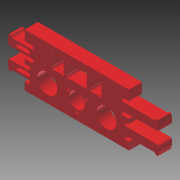
# Autodesk Inventor part: gantry6
Saved by Autodesk Inventor 2012 SP1 (Build 160190100, 190)
## iProperties
Created: 2011-10-14
Part Number: gantry6
Document SubType Name: Modeling
Designer: cramera
Density: 0.952 g/cm^3
Material: High Density Polyethylene
Mass: 43.3758 g
Surface Area: 190.421 cm^2
Volume: 45.5628 cm^3
Autodesk Inventor part; units mm, degrees
ref_plane "YZ Plane" through (0, 0, 0) normal (1, 0, 0) x (0, 1, 0)
ref_plane "XZ Plane" through (0, 0, 0) normal (0, 1, 0) x (-1, 0, 0)
ref_plane "XY Plane" through (0, 0, 0) normal (0, 0, 1) x (1, 0, 0)
derived "skeleton.ipt"
sketch "DRILL-THROUGH" plane through (0, 0, 0) normal (0, 0, 1) x (1, 0, 0)
  arc A0 (91.9322, 359.304) -> (93.4322, 360.804) centre (91.9322, 360.804) ccw
  arc A1 (93.4322, 360.804) -> (91.9322, 362.304) centre (91.9322, 360.804) ccw
  arc A2 (91.9322, 362.304) -> (90.4322, 360.804) centre (91.9322, 360.804) ccw
  arc A3 (90.4322, 360.804) -> (91.9322, 359.304) centre (91.9322, 360.804) ccw
  arc A4 (75.4345, 359.304) -> (76.9345, 360.804) centre (75.4345, 360.804) ccw
  arc A5 (76.9345, 360.804) -> (75.4345, 362.304) centre (75.4345, 360.804) ccw
  arc A6 (75.4345, 362.304) -> (73.9345, 360.804) centre (75.4345, 360.804) ccw
  arc A7 (73.9345, 360.804) -> (75.4345, 359.304) centre (75.4345, 360.804) ccw
  arc A8 (83.6834, 345.0165) -> (85.1834, 346.5165) centre (83.6834, 346.5165) ccw
  arc A9 (85.1834, 346.5165) -> (83.6834, 348.0165) centre (83.6834, 346.5165) ccw
  arc A10 (83.6834, 348.0165) -> (82.1834, 346.5165) centre (83.6834, 346.5165) ccw
  arc A11 (82.1834, 346.5165) -> (83.6834, 345.0165) centre (83.6834, 346.5165) ccw
  constraints: 24 point on circle, 12 centre point
sketch "STOCK_12MM" plane through (0, 0, 0) normal (0, 0, 1) x (1, 0, 0)
  line L0 (914.4, 914.4) -> (457.2, 914.4)
  line L1 (457.2, 914.4) -> (457.2, 0)
  line L2 (0, 0) -> (457.2, 0)
  line L3 (457.2, 0) -> (457.2, 914.4)
  line L4 (457.2, 914.4) -> (0, 914.4)
  line L5 (0, 914.4) -> (0, 0)
  line L6 (457.2, 0) -> (914.4, 0)
  line L7 (914.4, 0) -> (914.4, 914.4)
  constraints: 16 end point
sketch "THROUGH-CUT" plane through (0, 0, 0) normal (0, 0, 1) x (1, 0, 0)
  arc A0 (74.7934, 371.8768) -> (77.0384, 369.6317) centre (75.9159, 370.7543) ccw
  line L0 (77.0384, 369.6317) -> (90.3283, 369.6317)
  arc A1 (90.3283, 369.6317) -> (92.5734, 369.6317) centre (91.4508, 370.7543) ccw
  arc A2 (92.5734, 369.6317) -> (92.5734, 371.8768) centre (91.4508, 370.7543) ccw
  line L1 (92.5734, 371.8768) -> (92.5734, 379.7057)
  arc A3 (92.5734, 379.7057) -> (90.3283, 381.9507) centre (91.4508, 380.8282) ccw
  line L2 (90.3283, 381.9507) -> (77.0384, 381.9507)
  arc A4 (77.0384, 381.9507) -> (74.7934, 379.7057) centre (75.9159, 380.8282) ccw
  line L3 (74.7934, 379.7057) -> (74.7934, 371.8768)
  arc A5 (95.8754, 371.8768) -> (98.1204, 369.6317) centre (96.9979, 370.7543) ccw
  line L4 (98.1204, 369.6317) -> (103.7903, 369.6317)
  arc A6 (103.7903, 369.6317) -> (106.0354, 369.6317) centre (104.9128, 370.7543) ccw
  arc A7 (106.0354, 369.6317) -> (106.0354, 371.8768) centre (104.9128, 370.7543) ccw
  line L5 (106.0354, 371.8768) -> (106.0354, 379.7057)
  arc A8 (106.0354, 379.7057) -> (103.7903, 381.9507) centre (104.9128, 380.8282) ccw
  line L6 (103.7903, 381.9507) -> (98.1204, 381.9507)
  arc A9 (98.1204, 381.9507) -> (95.8754, 379.7057) centre (96.9979, 380.8282) ccw
  line L7 (95.8754, 379.7057) -> (95.8754, 371.8768)
  arc A10 (69.2463, 369.6317) -> (71.4914, 371.8768) centre (70.3688, 370.7543) ccw
  line L8 (71.4914, 371.8768) -> (71.4914, 379.7057)
  arc A11 (71.4914, 379.7057) -> (69.2463, 381.9507) centre (70.3688, 380.8282) ccw
  line L9 (69.2463, 381.9507) -> (63.5764, 381.9507)
  arc A12 (63.5764, 381.9507) -> (61.3314, 379.7057) centre (62.4539, 380.8282) ccw
  line L10 (61.3314, 379.7057) -> (61.3314, 371.8768)
  arc A13 (61.3314, 371.8768) -> (61.3314, 369.6317) centre (62.4539, 370.7543) ccw
  arc A14 (61.3314, 369.6317) -> (63.5764, 369.6317) centre (62.4539, 370.7543) ccw
  line L11 (63.5764, 369.6317) -> (69.2463, 369.6317)
  circle A15 centre (83.6834, 356.0415) radius 7.1882
  circle A16 centre (56.6971, 356.0411) radius 9.04
  circle A17 centre (110.6721, 356.0411) radius 9.04
  arc A18 (39.2334, 370.5512) -> (40.8209, 372.1387) centre (39.2334, 372.1387) ccw
  line L12 (40.8209, 372.1387) -> (40.8209, 372.2657)
  arc A19 (40.8209, 372.2657) -> (39.2334, 373.8532) centre (39.2334, 372.2657) ccw
  line L13 (39.2334, 373.8532) -> (29.2924, 373.8532)
  arc A20 (29.2924, 373.8532) -> (27.7049, 372.2657) centre (29.2924, 372.2657) ccw
  line L14 (27.7049, 372.2657) -> (27.7049, 372.1387)
  arc A21 (27.7049, 372.1387) -> (29.2924, 370.5512) centre (29.2924, 372.1387) ccw
  line L15 (29.2924, 370.5512) -> (39.2334, 370.5512)
  line L16 (131.3084, 350.4852) -> (154.7384, 350.4852)
  line L17 (154.7384, 350.4852) -> (156.0084, 348.9612)
  line L18 (156.0084, 348.9612) -> (157.7263, 348.9612)
  line L19 (157.7263, 348.9612) -> (158.5484, 352.5608)
  line L20 (158.5484, 352.5608) -> (158.5484, 356.2659)
  arc A22 (158.5484, 356.2659) -> (156.9609, 357.8512) centre (156.9609, 356.2637) ccw
  line L21 (156.9609, 357.8512) -> (128.1334, 357.8512)
  arc A23 (126.5459, 359.4387) -> (128.1334, 357.8512) centre (128.1334, 359.4387) ccw
  line L22 (126.5459, 359.4387) -> (126.5459, 359.5657)
  arc A24 (128.1334, 361.1532) -> (126.5459, 359.5657) centre (128.1334, 359.5657) ccw
  line L23 (128.1334, 361.1532) -> (131.3084, 361.1532)
  line L24 (131.3084, 361.1532) -> (131.3084, 365.2172)
  line L25 (131.3084, 365.2172) -> (124.9584, 365.2172)
  arc A25 (123.3709, 366.8047) -> (124.9584, 365.2172) centre (124.9584, 366.8047) ccw
  line L26 (123.3709, 366.8047) -> (123.3709, 366.9317)
  arc A26 (124.9584, 368.5192) -> (123.3709, 366.9317) centre (124.9584, 366.9317) ccw
  line L27 (124.9584, 368.5192) -> (156.9609, 368.5192)
  arc A27 (156.9609, 368.5192) -> (158.5484, 370.1045) centre (156.9609, 370.1067) ccw
  line L28 (158.5484, 370.1045) -> (158.5484, 373.8096)
  line L29 (158.5484, 373.8096) -> (157.7263, 377.4092)
  line L30 (157.7263, 377.4092) -> (156.0084, 377.4092)
  line L31 (156.0084, 377.4092) -> (154.7384, 375.8852)
  line L32 (154.7384, 375.8852) -> (131.3084, 375.8852)
  line L33 (131.3084, 375.8852) -> (124.9584, 375.8852)
  arc A28 (123.3709, 377.4727) -> (124.9584, 375.8852) centre (124.9584, 377.4727) ccw
  line L34 (123.3709, 377.4727) -> (123.3709, 377.5997)
  arc A29 (124.9584, 379.1872) -> (123.3709, 377.5997) centre (124.9584, 377.5997) ccw
  line L35 (124.9584, 379.1872) -> (131.3084, 379.1872)
  line L36 (131.3084, 379.1872) -> (131.3084, 388.3007)
  line L37 (131.3084, 388.3007) -> (36.0584, 388.3007)
  line L38 (36.0584, 388.3007) -> (36.0584, 379.1872)
  line L39 (36.0584, 379.1872) -> (42.4084, 379.1872)
  arc A30 (43.9959, 377.5997) -> (42.4084, 379.1872) centre (42.4084, 377.5997) ccw
  line L40 (43.9959, 377.5997) -> (43.9959, 377.4727)
  arc A31 (42.4084, 375.8852) -> (43.9959, 377.4727) centre (42.4084, 377.4727) ccw
  line L41 (42.4084, 375.8852) -> (36.0584, 375.8852)
  line L42 (36.0584, 375.8852) -> (27.2556, 375.8852)
  line L43 (27.2556, 375.8852) -> (24.6284, 375.8852)
  line L44 (24.6284, 375.8852) -> (23.3584, 377.4092)
  line L45 (23.3584, 377.4092) -> (21.6404, 377.4092)
  line L46 (21.6404, 377.4092) -> (20.8184, 373.8096)
  line L47 (20.8184, 373.8096) -> (20.8184, 370.1045)
  arc A32 (20.8184, 370.1045) -> (22.4059, 368.5192) centre (22.4059, 370.1067) ccw
  line L48 (22.4059, 368.5192) -> (36.0584, 368.5192)
  line L49 (36.0584, 368.5192) -> (42.4084, 368.5192)
  arc A33 (43.9959, 366.9317) -> (42.4084, 368.5192) centre (42.4084, 366.9317) ccw
  line L50 (43.9959, 366.9317) -> (43.9959, 366.8047)
  arc A34 (42.4084, 365.2172) -> (43.9959, 366.8047) centre (42.4084, 366.8047) ccw
  line L51 (42.4084, 365.2172) -> (36.0584, 365.2172)
  line L52 (36.0584, 365.2172) -> (36.0584, 361.1532)
  line L53 (36.0584, 361.1532) -> (39.2334, 361.1532)
  arc A35 (40.8209, 359.5657) -> (39.2334, 361.1532) centre (39.2334, 359.5657) ccw
  line L54 (40.8209, 359.5657) -> (40.8209, 359.4387)
  arc A36 (39.2334, 357.8512) -> (40.8209, 359.4387) centre (39.2334, 359.4387) ccw
  line L55 (39.2334, 357.8512) -> (36.0584, 357.8512)
  line L56 (36.0584, 357.8512) -> (22.4059, 357.8512)
  arc A37 (22.4059, 357.8512) -> (20.8184, 356.2659) centre (22.4059, 356.2637) ccw
  line L57 (20.8184, 356.2659) -> (20.8184, 352.5608)
  line L58 (20.8184, 352.5608) -> (21.6404, 348.9612)
  line L59 (21.6404, 348.9612) -> (23.3584, 348.9612)
  line L60 (23.3584, 348.9612) -> (24.6284, 350.4852)
  line L61 (24.6284, 350.4852) -> (27.2556, 350.4852)
  line L62 (27.2556, 350.4852) -> (36.0584, 350.4852)
  line L63 (36.0584, 350.4852) -> (39.2334, 350.4852)
  arc A38 (40.8209, 348.8977) -> (39.2334, 350.4852) centre (39.2334, 348.8977) ccw
  line L64 (40.8209, 348.8977) -> (40.8209, 348.7707)
  arc A39 (39.2334, 347.1832) -> (40.8209, 348.7707) centre (39.2334, 348.7707) ccw
  line L65 (39.2334, 347.1832) -> (36.0584, 347.1832)
  line L66 (36.0584, 347.1832) -> (36.0584, 340.1665)
  line L67 (36.0584, 340.1665) -> (131.3084, 340.1665)
  line L68 (131.3084, 340.1665) -> (131.3084, 347.1832)
  line L69 (131.3084, 347.1832) -> (128.1334, 347.1832)
  arc A40 (126.5459, 348.7707) -> (128.1334, 347.1832) centre (128.1334, 348.7707) ccw
  line L70 (126.5459, 348.7707) -> (126.5459, 348.8977)
  arc A41 (128.1334, 350.4852) -> (126.5459, 348.8977) centre (128.1334, 348.8977) ccw
  line L71 (128.1334, 350.4852) -> (131.3084, 350.4852)
  arc A42 (29.3049, 355.8192) -> (27.7174, 354.2317) centre (29.3049, 354.2317) ccw
  line L72 (27.7174, 354.2317) -> (27.7049, 354.1047)
  arc A43 (27.7049, 354.1047) -> (29.2924, 352.5172) centre (29.2924, 354.1047) ccw
  line L73 (29.2924, 352.5172) -> (39.2334, 352.5172)
  arc A44 (39.2334, 352.5172) -> (40.8209, 354.1047) centre (39.2334, 354.1047) ccw
  line L74 (40.8209, 354.1047) -> (40.8209, 354.2317)
  arc A45 (40.8209, 354.2317) -> (39.2334, 355.8192) centre (39.2334, 354.2317) ccw
  line L75 (39.2334, 355.8192) -> (29.3049, 355.8192)
  dimension "d5" = 18.08
  dimension "d6" = 18.08
  dimension "d7" = 53.975
  constraints: 152 end point, 86 point on circle, 46 centre point
  measures "d5" diameter of A16
  measures "d6" diameter of A17
  measures "d7" distance of A17.centre A16.centre
extrude "Extrusion1" add sketch "THROUGH-CUT" along normal blind 12
extrude "Extrusion2" cut sketch "DRILL-THROUGH" along normal through all
equation "\"d6\" = d5"
equation "\"d1\" = StockThickness"
equation "\"StockThickness\" = 12"
body "Solid1"
